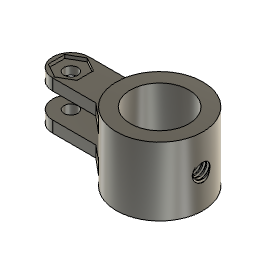
Mount for Half Inch Rod Parallel v6 (Autodesk Fusion 360 design; units mm, degrees)
Autodesk Fusion 360 part; units mm, degrees
sketch "Sketch1" plane through (0, 0, 0) normal (0, 0, 1) x (1, 0, 0)
  circle A0 centre (0, 0) radius 6.425
  circle A1 centre (0, 0) radius 9.5
  dimension "d28" = 12.85
  dimension "d29" = 19
  constraint coincident A0.centre A1.centre
  measures "d28" diameter of A0
  measures "d29" diameter of A1
sketch "Sketch2" plane through (0, 0, 0) normal (0, 0, 1) x (1, 0, 0)
  line L0 (0, 0) -> (-20, 0)
  constraint coincident L0.start origin
  constraint horizontal L0
sketch "Sketch3" plane through (0, 0, 0) normal (0, 0, 1) x (1, 0, 0)
  line L0 (0, 0) -> (-9.5, 0)
  line L1 (-9.5, 0) -> (-19.5, 0)
  circle A0 centre (-19.5, 0) radius 1.5025
  arc A1 (-19.5, 4) -> (-19.5, -4) centre (-19.5, 0) ccw
  line L2 (-19.5, 4) -> (-10, 4)
  line L3 (-19.5, -4) -> (-10, -4)
  line L4 (-10, -4) -> (-6.25, -7.15)
  line L5 (-6.25, 7.15) -> (-10, 4)
  line L6 (-6.25, -7.15) -> (-8, 0)
  line L7 (-8, 0) -> (-6.25, 7.15)
  dimension "d30" = 9.5
  dimension "d31" = 10
  dimension "d32" = 3.005
  dimension "d33" = 4
  dimension "d34" = 14.3
  constraint coincident L0.start origin
  constraint horizontal L0
  constraint parallel L0 L1
  constraint coincident L1.end A0.centre
  constraint tangent A1 L2
  constraint horizontal L2
  constraint tangent A1 L3
  constraint horizontal L3
  constraint coincident L0 L6.end
  measures "d30" distance of L0.start L0.end
  measures "d31" distance of L0.end L1.end
  measures "d32" diameter of A0
  measures "d33" radius of A1
  measures "d34" distance of L4.end L5.start
extrude "Extrude1" add sketch "Sketch1" along normal mid plane 15 makes body 1
hole "Hole1" at (9.5, 0, -0.0147) direction (-1, 0, 0) diameter 3.416 depth 5 tip angle 180 bodies 1
thread "Thread1" "ANSI Unified Screw Threads 0.164(#8) 8-32 UNC 2B"
extrude "Extrude4" add sketch "Sketch3" along normal blind 2.5 from surface at 2.753 bodies 1
extrude "Extrude5" add sketch "Sketch3" against normal blind 2.5 from surface at -2.753 bodies 1
sketch "Sketch4" plane through (0, 0, 0) normal (0, 0, 1) x (1, 0, 0)
  line L0 (-16.3755, 1.8098) -> (-19.5051, 3.6107)
  line L1 (-19.5051, 3.6107) -> (-22.6295, 1.801)
  line L2 (-22.6295, 1.801) -> (-22.6245, -1.8098)
  line L3 (-22.6245, -1.8098) -> (-19.4949, -3.6107)
  line L4 (-19.4949, -3.6107) -> (-16.3705, -1.801)
  line L5 (-16.3705, -1.801) -> (-16.3755, 1.8098)
  point P0 (-20, 0)
  point P1 (-19.5, 0)
  dimension "d35" = 3.127
  measures "d35" distance of P1 L5
extrude "Extrude6" cut sketch "Sketch4" along normal blind 0.753 from surface at 4.5 bodies 1
thread "Thread2" "ANSI Unified Screw Threads 0.164(#8) 8-32 UNC 2B" major diameter 4.1656 minor diameter 3.4163 pitch 0.7937 angle 60 modelled right hand crest width 0.2341 on face at (8.4537, 0.5924, -1.6167) crest through (9.302, 1.7082, -0.0147) on bodies 1
copy_body "Body->Comp1" bodies 1 removing the originals makes body 2 in component "Component"
component "Component" placed x (1, 0, 0) y (0, 1, 0) z (0, 0, 1) at (0, 0, 0)
component "V2" placed x (1, 0, 0) y (0, 1, 0) z (0, 0, 1) at (0, 0, 0)
named bodies: "Sleeve Camera Mount 1"
